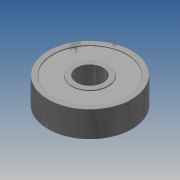
# Autodesk Inventor part: Kugellager625_5x16x5
Saved by Autodesk Inventor 2015 (Build 190159000, 159)
## iProperties
Created: 2015-01-08
Part Number: Kugellager625_5x16x5
Material: Stahl, Kohlenstoff
Document SubType Name: Modeling
Designer: Marc
Mass: 1.75158 g
Surface Area: 3.19634 cm^2
Volume: 0.223132 cm^3
Density: 7.85 g/cm^3
Appearance: Halbpoliert
Author: Marc
Autodesk Inventor part; units mm, degrees
ref_plane "YZ Plane" through (0, 0, 0) normal (1, 0, 0) x (0, 1, 0)
ref_plane "XZ Plane" through (0, 0, 0) normal (0, 1, 0) x (-1, 0, 0)
ref_plane "XY Plane" through (0, 0, 0) normal (0, 0, 1) x (1, 0, 0)
sketch "Skizze1" plane through (0, 0, 0) normal (0, 0, 1) x (1, 0, 0)
  line L0 (-11.2, 0) -> (11.2, 0) projected
  line L1 (0, -11.2) -> (0, 11.2) projected
  circle A0 centre (0, 0) radius 8
  circle A1 centre (0, 0) radius 2.5
  dimension "d0" = 16
  dimension "d1" = 5
  constraints: 2 centre point, 2 coincident
  measures "d0" diameter of A0
  measures "d1" diameter of A1
extrude "Extrusion1" add sketch "Skizze1" along normal mid plane 5 contours A1 L1 A0 L0 | L0 A0 L1 A1 | A1 L0 A0 L1 | L1 A0 L0 A1
sketch "Skizze2" plane through (0, 0, 2.5) normal (0, 0, 1) x (1, 0, 0)
  circle A0 centre (0, 0) radius 2.5 projected
  circle A1 centre (0, 0) radius 8 projected
  circle A2 centre (0, 0) radius 3.5
  circle A3 centre (0, 0) radius 7
  dimension "d4" = 7
  dimension "d5" = 14
  constraints: 2 centre point, 2 coincident
  measures "d4" diameter of A2
  measures "d5" diameter of A3
extrude "Extrusion2" cut sketch "Skizze2" against normal blind 0.2 contours A3
mirror "Spiegeln1" about plane through (0, 0, 0) normal (0, 0, 1) of "Extrusion2"
chamfer "Fase1" distance 0.05 angle 45 1 edges at (-7, 0, 2.5)
chamfer "Fase2" distance 0.05 angle 45 1 edges at (-3.5, 0, 2.5)
chamfer "Fase3" distance 0.05 angle 45 1 edges at (-2.5, 0, 2.5)
chamfer "Fase4" distance 0.05 angle 45 1 edges at (-8, 0, 2.5)
chamfer "Fase5" distance 0.05 angle 45 1 edges at (-8, 0, -2.5)
chamfer "Fase6" distance 0.05 angle 45 1 edges at (-7, 0, -2.5)
chamfer "Fase7" distance 0.05 angle 45 1 edges at (-3.5, 0, -2.5)
chamfer "Fase8" distance 0.05 angle 45 1 edges at (-2.5, 0, -2.5)
